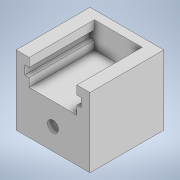
# Autodesk Inventor part: usb port mount
Saved by Autodesk Inventor 2020.3 (Build 243373000, 373)
## iProperties
Created: 2020-08-21
Part Number: usb port mount
Material: Generic
Document SubType Name: Modeling
Designer: joesp
Density: 1 g/cm^3
Appearance: Default
Author: joesp
Autodesk Inventor part; units mm, degrees
ref_plane "YZ Plane" through (0, 0, 0) normal (1, 0, 0) x (0, 1, 0)
ref_plane "XZ Plane" through (0, 0, 0) normal (0, 1, 0) x (-1, 0, 0)
ref_plane "XY Plane" through (0, 0, 0) normal (0, 0, 1) x (1, 0, 0)
sketch "Sketch1" plane through (0, 0, 0) normal (0, 0, 1) x (1, 0, 0)
  line L0 (0, 0) -> (-17, 0)
  line L1 (-17, 0) -> (-17, -10)
  line L2 (-17, -10) -> (0, -10)
  line L3 (0, -10) -> (0, 0)
  line L4 (-17, 0) -> (-14, 0)
  line L5 (-14, 0) -> (-14, 6)
  line L6 (-14, 6) -> (-17, 6)
  line L7 (-17, 6) -> (-17, 0)
  line L8 (-14, 4) -> (-15, 4)
  line L9 (-15, 4) -> (-15, 2)
  line L10 (-15, 2) -> (-14, 2)
  line L11 (-14, 2) -> (-14, 4)
  line L12 (0, 0) -> (-3, 0)
  line L13 (-3, 0) -> (-3, 6)
  line L14 (-3, 6) -> (0, 6)
  line L15 (0, 6) -> (0, 0)
  line L16 (-3, 4) -> (-2, 4)
  line L17 (-2, 4) -> (-2, 2)
  line L18 (-2, 2) -> (-3, 2)
  line L19 (-3, 2) -> (-3, 4)
  dimension "d1" = 10
  dimension "d10" = 13
  dimension "d11" = 2
  dimension "d12" = 2
  dimension "d13" = 2
  dimension "d14" = 2
  dimension "d15" = 2
  dimension "d16" = 1
  dimension "d17" = 1
  constraints: 40 end point, 10 parallel, 5 horizontal, 5 perpendicular, 5 point on line
  measures "d1" distance of L0.end L1.end
  measures "d10" distance between parallel lines of L17 L9
  measures "d11" distance between parallel lines of L15 L17
  measures "d12" distance between parallel lines of L0 L10
  measures "d13" distance between parallel lines of L6 L8
  measures "d14" distance of L8.end L9.end
  measures "d15" distance between parallel lines of L7 L9
  measures "d16" distance of L9.end L10.end
  measures "d17" distance of L17.end L18.end
extrude "Extrusion1" add sketch "Sketch1" along normal blind 15 contours L3 L2 L1 L0 | L0 L13 L18 L17 L16 L14 L15 | L0 L7 L6 L5 L8 L9 L10
sketch "Sketch2" plane through (0, 0, 15) normal (0, 0, 1) x (1, 0, 0)
  circle A0 centre (-8.5, -5) radius 1.25
  line L0 (0, 0) -> (-14, 0) projected
  point P0 (-17, 0)
  point P1 (-8.5, 0)
  dimension "d4" = 5
  dimension "d5" = 2.5
  constraints: 1 centre point, 1 point on line, 1 vertical alignment
  measures "d4" distance from line of L0 A0.centre
  measures "d5" diameter of A0
sketch "Sketch4" plane through (0, 0, 0) normal (0, 0, -1) x (-1, 0, 0)
  line L0 (0, -10) -> (0, 6) projected
  line L1 (17, 6) -> (17, -10) projected
  line L2 (0, -10) -> (17, -10)
  line L3 (17, -10) -> (17, 6)
  line L4 (17, 6) -> (0, 6)
  line L5 (0, 6) -> (0, -10)
  point P0 (0, 0)
  point P1 (0, 6)
  constraints: 8 end point, 2 parallel, 1 horizontal, 1 perpendicular
extrude "Extrusion3" add sketch "Sketch4" along normal blind 2
extrude "Extrusion4" cut sketch "Sketch2" against normal through all
equation "\"d15\" = d11"
equation "\"d16\" = d17"
body "Solid1"
